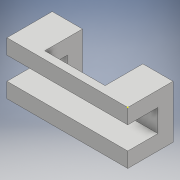
# Autodesk Inventor part: P3-13
Saved by Autodesk Inventor 2017 (Build 210142000, 142)
## iProperties
Created: 2017-02-13
Part Number: P3-13
Material: Generic
Document SubType Name: Modeling
Designer: Schaffel
Density: 1 g/cm^3
Appearance: Default
Author: Schaffel
Autodesk Inventor part; units mm, degrees
ref_plane "YZ Plane" through (0, 0, 0) normal (1, 0, 0) x (0, 1, 0)
ref_plane "XZ Plane" through (0, 0, 0) normal (0, 1, 0) x (-1, 0, 0)
ref_plane "XY Plane" through (0, 0, 0) normal (0, 0, 1) x (1, 0, 0)
sketch "Sketch1" plane through (0, 0, 0) normal (0, 0, 1) x (1, 0, 0)
  point P0 (0, 0)
sketch "Sketch2" plane through (0, 0, 0) normal (1, 0, 0) x (0, 1, 0)
  line L0 (0, 0) -> (30, 0)
  line L1 (30, 0) -> (30, -35)
  line L2 (30, -35) -> (0, -35)
  line L3 (0, -35) -> (0, -25)
  line L4 (0, -25) -> (20, -25)
  line L5 (20, -25) -> (20, -10)
  line L6 (20, -10) -> (0, -10)
  line L7 (0, -10) -> (0, 0)
  constraints: 16 end point, 7 perpendicular, 1 horizontal, 1 point on line
extrude "Extrusion1" add sketch "Sketch2" against normal blind 20
sketch "Sketch3" plane through (-20, 0, 0) normal (-1, 0, 0) x (0, 0, 1)
  line L0 (0, 0) -> (0, 30) projected
  line L1 (0, 5) -> (0, 0)
  line L2 (-35, 30) -> (-35, 0) projected
  line L3 (-35, 30) -> (-35, 25)
  line L4 (-35, 25) -> (0, 5)
  line L5 (-35, 25) -> (-35, 0)
  line L6 (-35, 0) -> (-25, 0) projected
  line L7 (-35, 0) -> (-25, 0)
  line L8 (-25, 0) -> (-25, 19.2857)
  line L9 (-25, 0) -> (-25, 20) projected
  line L10 (-25, 19.2857) -> (-35, 25)
  line L11 (-10, 20) -> (-10, 0) projected
  line L12 (-10, 10.7143) -> (0, 5)
  line L13 (-10, 0) -> (0, 0) projected
  line L14 (0, 0) -> (-10, 0)
  line L15 (-10, 0) -> (-10, 10.7143)
  constraints: 20 end point, 8 point on line, 3 collinear, 1 parallel, 1 perpendicular, 1 vertical
extrude "Extrusion2" add sketch "Sketch3" along normal blind 40
sketch "Sketch4" plane through (-60, 0, 0) normal (-1, 0, 0) x (0, 0, 1)
  line L0 (-35, 25) -> (-35, 0) projected
  line L1 (-35, 0) -> (-35, 30)
  line L2 (0, 30) -> (-35, 30) projected
  line L3 (-35, 30) -> (0, 30)
  line L4 (0, 0) -> (0, 30) projected
  line L5 (0, 30) -> (0, 0)
  line L6 (0, 0) -> (-10, 0)
  line L7 (-25, 20) -> (-10, 20) projected
  line L8 (-10, 0) -> (-10, 20)
  line L9 (-25, 0) -> (-25, 20) projected
  line L10 (-10, 20) -> (-25, 20)
  line L11 (-25, 20) -> (-25, 0)
  line L12 (-25, 0) -> (-35, 0)
  constraints: 16 end point, 4 collinear, 4 perpendicular
extrude "Extrusion3" add sketch "Sketch4" along normal blind 20
body "Solid1"
